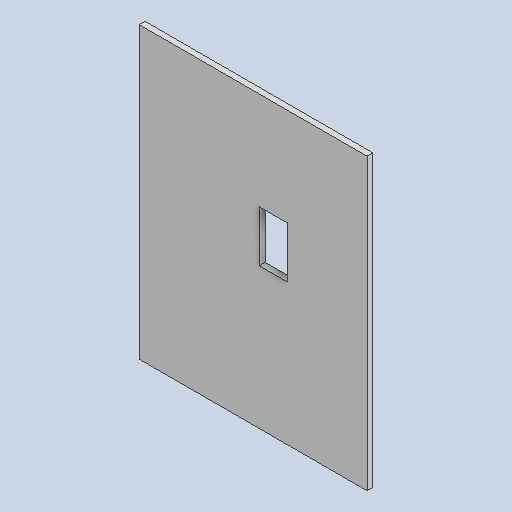
# Autodesk Inventor part: przod
Saved by Autodesk Inventor 2022 (Build 260153000, 153)
## iProperties
Created: 2023-01-18
Part Number: przod
Material: Generic
Document SubType Name: Modeling
Designer: komputer
Density: 1 g/cm^3
Appearance: Default
Author: komputer
Autodesk Inventor part; units mm, degrees
ref_plane "YZ Plane" through (0, 0, 0) normal (1, 0, 0) x (0, 1, 0)
ref_plane "XZ Plane" through (0, 0, 0) normal (0, 1, 0) x (-1, 0, 0)
ref_plane "XY Plane" through (0, 0, 0) normal (0, 0, 1) x (1, 0, 0)
sketch "Sketch1" plane through (0, 0, 0) normal (0, 0, 1) x (1, 0, 0)
  line L0 (9.1023, -3.4337) -> (9.1023, 0.9663) projected
  line L1 (6.7023, -3.4337) -> (9.1023, -3.4337) projected
  line L2 (6.7023, 0.9663) -> (6.7023, -3.4337) projected
  line L3 (9.1023, 0.9663) -> (6.7023, 0.9663) projected
  line L4 (-3.672, 5.3) -> (-3.672, 9.4)
  line L5 (17.5929, 9.4) -> (17.5929, -15.6) projected
  line L6 (17.5929, -15.6) -> (-3.672, -15.6)
  line L7 (-3.672, -15.6) -> (-3.672, 9.4)
  line L8 (-3.672, 9.4) -> (17.5929, 9.4)
  line L9 (17.5929, 9.4) -> (17.5929, -15.6)
  point P0 (0, 0)
  constraints: 10 end point, 2 parallel, 1 horizontal, 1 perpendicular, 1 vertical, 2 other
extrude "Extrusion1" add sketch "Sketch1" along normal blind 0.7
sketch "Sketch2" plane through (0, 0, 0) normal (0, 0, -1) x (-1, 0, 0)
  line L0 (-17.5929, -15.6) -> (-17.5929, 9.4) projected
  line L1 (3.672, -15.6) -> (-17.5929, -15.6) projected
  line L2 (3.672, 9.4) -> (3.672, -15.6) projected
  line L3 (-17.5929, 9.4) -> (3.672, 9.4) projected
  line L4 (-9.1023, -3.4337) -> (-6.7023, -3.4337) projected
  line L5 (-9.1023, 0.9663) -> (-9.1023, -3.4337) projected
  line L6 (-6.7023, 0.9663) -> (-9.1023, 0.9663) projected
  line L7 (-6.7023, -3.4337) -> (-6.7023, 0.9663) projected
  point P0 (0, 0)
extrude "Extrusion2" cut sketch "Sketch2" against normal blind 0.2
sketch "Sketch3" plane through (0, 0, 0.7) normal (0, 0, 1) x (1, 0, 0)
  line L0 (15.9929, 9.4) -> (15.9929, -15.6) projected
  line L1 (15.9929, -15.6) -> (17.5929, -15.6) projected
  line L2 (17.5929, 9.4) -> (17.5929, -15.6) projected
  line L3 (15.9929, 9.4) -> (17.5929, 9.4) projected
  point P0 (0, 0)
extrude "Extrusion3" cut sketch "Sketch3" against normal through all
body "Solid1"
